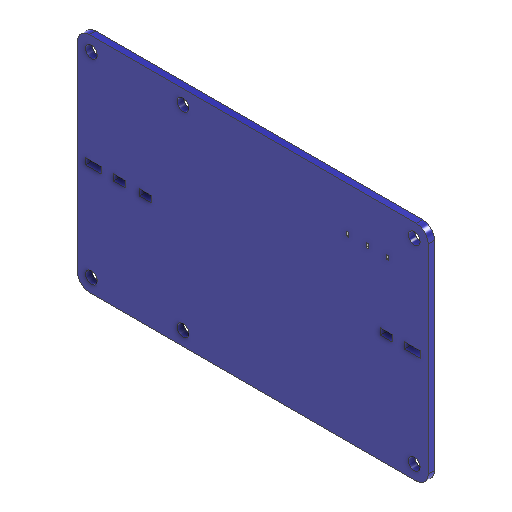
# Autodesk Inventor part: PCB_1
Saved by Autodesk Inventor 2025.2 (Build 292293000, 293)
## iProperties
Created: 2025-03-09
Part Number: PCB_1
Material: Generic
Document SubType Name: Modeling
Designer: ahorat
Density: 1 g/cm^3
Appearance: Default
Author: ahorat
Autodesk Inventor part; units mm, degrees
ref_plane "YZ Plane" through (0, 0, 0) normal (1, 0, 0) x (0, 1, 0)
ref_plane "XZ Plane" through (0, 0, 0) normal (0, 1, 0) x (-1, 0, 0)
ref_plane "XY Plane" through (0, 0, 0) normal (0, 0, 1) x (1, 0, 0)
sketch "Sketch1" plane through (0, 0, 0) normal (0, 0, 1) x (1, 0, 0)
  line L0 (-41, -28) -> (41, -28)
  line L1 (44, -25) -> (44, 25)
  line L2 (41, 28) -> (-41, 28)
  line L3 (-44, 25) -> (-44, -25)
  line L4 (-44, -28) -> (44, 28) construction
  line L5 (44, -28) -> (-44, 28) construction
  arc A0 (-41, 28) -> (-44, 25) centre (-41, 25) ccw
  arc A1 (44, 25) -> (41, 28) centre (41, 25) ccw
  arc A2 (41, -28) -> (44, -25) centre (41, -25) ccw
  arc A3 (-44, -25) -> (-41, -28) centre (-41, -25) ccw
  point P0 (0, 0)
  dimension "d0" = 88
  dimension "d1" = 56
  dimension "d2" = 3
  constraints: 12 end point, 8 point on circle, 8 point on line, 8 tangent, 4 centre point, 3 equal radius, 2 midpoint, 2 parallel, 1 horizontal, 1 perpendicular
  measures "d0" distance of L4.end L5.end
  measures "d1" distance of L5.end L4.start
  measures "d2" radius of A0
extrude "Extrusion1" add sketch "Sketch1" along normal blind 1.6
sketch "Sketch2" plane through (0, 0, 1.6) normal (0, 0, 1) x (1, 0, 0)
  line L0 (-42, -0.8) -> (-38, -0.8)
  line L1 (-38, -0.8) -> (-38, 0.8)
  line L2 (-38, 0.8) -> (-42, 0.8)
  line L3 (-42, 0.8) -> (-42, -0.8)
  line L4 (-42, -0.8) -> (-38, 0.8) construction
  line L5 (-38, -0.8) -> (-42, 0.8) construction
  line L6 (-35, -0.8) -> (-32, -0.8)
  line L7 (-32, -0.8) -> (-32, 0.8)
  line L8 (-32, 0.8) -> (-35, 0.8)
  line L9 (-35, 0.8) -> (-35, -0.8)
  line L10 (-35, -0.8) -> (-32, 0.8) construction
  line L11 (-32, -0.8) -> (-35, 0.8) construction
  line L12 (-28.5, -0.8) -> (-25.5, -0.8)
  line L13 (-25.5, -0.8) -> (-25.5, 0.8)
  line L14 (-25.5, 0.8) -> (-28.5, 0.8)
  line L15 (-28.5, 0.8) -> (-28.5, -0.8)
  line L16 (-28.5, -0.8) -> (-25.5, 0.8) construction
  line L17 (-25.5, -0.8) -> (-28.5, 0.8) construction
  line L18 (32, -0.8) -> (35, -0.8)
  line L19 (35, -0.8) -> (35, 0.8)
  line L20 (35, 0.8) -> (32, 0.8)
  line L21 (32, 0.8) -> (32, -0.8)
  line L22 (32, -0.8) -> (35, 0.8) construction
  line L23 (35, -0.8) -> (32, 0.8) construction
  line L24 (38, -0.8) -> (42, -0.8)
  line L25 (42, -0.8) -> (42, 0.8)
  line L26 (42, 0.8) -> (38, 0.8)
  line L27 (38, 0.8) -> (38, -0.8)
  line L28 (38, -0.8) -> (42, 0.8) construction
  line L29 (42, -0.8) -> (38, 0.8) construction
  line L30 (-44, 25) -> (-44, -25) projected
  line L31 (44, -25) -> (44, 25) projected
  point P0 (0, 0)
  point P1 (-40, 0)
  point P2 (-33.5, 0)
  point P3 (-27, 0)
  point P4 (33.5, 0)
  point P5 (40, 0)
  dimension "d5" = 2
  dimension "d6" = 4
  dimension "d7" = 3
  dimension "d8" = 3
  dimension "d9" = 3.5
  dimension "d10" = 2
  dimension "d11" = 4
  dimension "d12" = 3
  dimension "d13" = 3
  dimension "d14" = 1.6
  constraints: 60 end point, 10 midpoint, 10 parallel, 5 horizontal, 5 horizontal alignment, 5 perpendicular, 4 point on line, 1 collinear
  measures "d5" distance between parallel lines of L30 L3
  measures "d6" distance of L1.end L2.end
  measures "d7" distance between parallel lines of L9 L1
  measures "d8" distance of L7.end L8.end
  measures "d9" distance between parallel lines of L15 L7
  measures "d10" distance between parallel lines of L31 L25
  measures "d11" distance of L25.end L26.end
  measures "d12" distance between parallel lines of L19 L27
  measures "d13" distance of L19.end L20.end
  measures "d14" distance of L2.end L0.start
extrude "Extrusion2" cut sketch "Sketch2" against normal blind 1.6
sketch "Sketch3" plane through (0, 0, 1.6) normal (0, 0, 1) x (1, 0, 0)
  line L0 (-40.5, 24.5) -> (-17.5, 24.5)
  line L1 (-17.5, 24.5) -> (-17.5, -24.5)
  line L2 (-17.5, -24.5) -> (-40.5, -24.5)
  line L3 (-40.5, -24.5) -> (-40.5, 24.5)
  line L4 (-17.5, 24.5) -> (40.5, 24.5)
  line L5 (40.5, 24.5) -> (40.5, -24.5)
  line L6 (40.5, -24.5) -> (-17.5, -24.5)
  line L7 (-44, 25) -> (-44, -25) projected
  point P0 (0, 0)
  point P1 (-40.5, 0)
  point P2 (-44, 0)
  dimension "d24" = 58
  dimension "d25" = 23
  dimension "d26" = 49
  dimension "d27" = 3.5
  constraints: 14 end point, 3 horizontal, 2 coincident, 2 midpoint, 2 parallel, 1 horizontal alignment, 1 perpendicular, 1 vertical
  measures "d24" distance of L0.end L4.end
  measures "d25" distance of L0.start L0.end
  measures "d26" distance of L4.end L5.end
  measures "d27" distance between parallel lines of L7 L3
hole "Hole1" at (-40.5, -24.5, 1.6) at (-17.5, -24.5, 1.6) at (40.5, -24.5, 1.6) at (40.5, 24.5, 1.6) at (-17.5, 24.5, 1.6) at (-40.5, 24.5, 1.6) direction (0, 0, -1) diameter 3 end through all
sketch "Sketch4" plane through (0, 0, 1.6) normal (0, 0, 1) x (1, 0, 0)
  line L0 (23.5, 16.5) -> (24, 16.5)
  line L1 (24, 16.5) -> (24, 17.5)
  line L2 (24, 17.5) -> (23.5, 17.5)
  line L3 (23.5, 17.5) -> (23.5, 16.5)
  line L4 (33.5, 16.5) -> (34, 16.5)
  line L5 (34, 16.5) -> (34, 17.5)
  line L6 (34, 17.5) -> (33.5, 17.5)
  line L7 (33.5, 17.5) -> (33.5, 16.5)
  line L8 (28.5, 16.5) -> (29, 16.5)
  line L9 (29, 16.5) -> (29, 17.5)
  line L10 (29, 17.5) -> (28.5, 17.5)
  line L11 (28.5, 17.5) -> (28.5, 16.5)
  line L12 (41, 28) -> (-41, 28) projected
  line L13 (44, -25) -> (44, 25) projected
  point P0 (0, 0)
  point P1 (28.75, 16.5)
  point P2 (23.75, 16.5)
  point P3 (33.75, 16.5)
  point P4 (34, 17)
  dimension "d28" = 0.5
  dimension "d29" = 5
  dimension "d30" = 5
  dimension "d31" = 11.5
  dimension "d32" = 1
  dimension "d33" = 10
  constraints: 24 end point, 6 parallel, 4 midpoint, 4 point on line, 3 horizontal, 3 perpendicular, 2 collinear
  measures "d28" distance of L1.end L2.end
  measures "d29" distance of point (28.75, 16.5) point (23.75, 16.5)
  measures "d30" distance of point (33.75, 16.5) point (28.75, 16.5)
  measures "d31" distance from line of L12 point (33.75, 16.5)
  measures "d32" distance of L4.end L5.end
  measures "d33" distance from line of L13 point (34, 17)
extrude "Extrusion3" cut sketch "Sketch4" against normal through all
body "Solid1"
